Autodesk Fusion 360 part; units mm, degrees
note: some values were not read from the file. Set by a fixed rule: which face or edge a step refers to.
(part 5 of 20)
  spline S25 degree 5 poles (11.0419, -11.5792) (11.0412, -11.5772) (11.0398, -11.5731) (11.0377, -11.5671) (11.035, -11.5591) (11.0315, -11.5491) (11.028, -11.5391) (11.0246, -11.5291) (11.0211, -11.5192) (11.0176, -11.5093) (11.0141, -11.4995) (11.0106, -11.4897) (11.0071, -11.4799) (11.0036, -11.4701) (11.0001, -11.4604) (10.9966, -11.4507) (10.993, -11.441) (10.9895, -11.4313) (10.986, -11.4217) (10.9824, -11.4122) (10.9789, -11.4026) (10.9753, -11.3931) (10.9717, -11.3836) (10.9682, -11.3742) (10.9646, -11.3647) (10.961, -11.3553) (10.9574, -11.346) (10.9538, -11.3367) (10.9502, -11.3274) (10.9466, -11.3181) (10.943, -11.3089) (10.9394, -11.2997) (10.9358, -11.2905) (10.9321, -11.2814) (10.9285, -11.2723) (10.9249, -11.2632) (10.9212, -11.2541) (10.9176, -11.2451) (10.9139, -11.2362) (10.9103, -11.2272) (10.9066, -11.2183) (10.903, -11.2094) (10.8993, -11.2006) (10.8957, -11.1918) (10.892, -11.183) (10.8883, -11.1743) (10.8847, -11.1655) (10.881, -11.1569) (10.8773, -11.1482) (10.8736, -11.1396) (10.8699, -11.131) (10.8662, -11.1225) (10.8625, -11.114) (10.8589, -11.1055) (10.8552, -11.097) (10.8515, -11.0886) (10.8478, -11.0803) (10.8441, -11.0719) (10.8404, -11.0636) (10.8367, -11.0553) (10.833, -11.0471) (10.8292, -11.0389) (10.8255, -11.0307) (10.8218, -11.0226) (10.8181, -11.0145) (10.8144, -11.0064) (10.8107, -10.9984) (10.807, -10.9903) (10.8033, -10.9824) (10.7996, -10.9745) (10.7958, -10.9666) (10.7921, -10.9587) (10.7884, -10.9509) (10.7847, -10.9431) (10.781, -10.9353) (10.7773, -10.9276) (10.7736, -10.9199) (10.7699, -10.9123) (10.7662, -10.9046) (10.7625, -10.8971) (10.7587, -10.8895) (10.755, -10.882) (10.7513, -10.8745) (10.7476, -10.8671) (10.7439, -10.8597) (10.7402, -10.8523) (10.7365, -10.845) (10.7328, -10.8377) (10.7292, -10.8305) (10.7255, -10.8233) (10.7218, -10.8161) (10.7181, -10.8089) (10.7144, -10.8018) (10.7107, -10.7947) (10.7071, -10.7877) (10.7034, -10.7807) (10.6997, -10.7738) (10.6961, -10.7668) (10.6924, -10.7599) (10.6888, -10.7531) (10.6851, -10.7463) (10.6815, -10.7395) (10.6778, -10.7328) (10.6742, -10.7261) (10.6706, -10.7194) (10.6669, -10.7128) (10.6633, -10.7062) (10.6597, -10.6997) (10.6561, -10.6931) (10.6525, -10.6867) (10.6489, -10.6802) (10.6453, -10.6738) (10.6417, -10.6675) (10.6381, -10.6612) (10.6346, -10.6549) (10.631, -10.6487) (10.6275, -10.6425) (10.6239, -10.6363) (10.6204, -10.6302) (10.6168, -10.6241) (10.6133, -10.618) (10.6098, -10.612) (10.6063, -10.6061) (10.6028, -10.6001) (10.5993, -10.5943) (10.5958, -10.5884) (10.5923, -10.5826) (10.5889, -10.5768) (10.5854, -10.5711) (10.582, -10.5654) (10.5785, -10.5598) (10.5751, -10.5542) (10.5717, -10.5486) (10.5683, -10.5431) (10.5649, -10.5376) (10.5615, -10.5321) (10.5582, -10.5267) (10.5548, -10.5214) (10.5515, -10.516) (10.5481, -10.5108) (10.5448, -10.5055) (10.5415, -10.5003) (10.5382, -10.4952) (10.5349, -10.4901) (10.5316, -10.485) (10.5284, -10.48) (10.5251, -10.475) (10.5219, -10.47) (10.5187, -10.4651) (10.5155, -10.4603) (10.5123, -10.4554) (10.5091, -10.4507) (10.506, -10.4459) (10.5028, -10.4412) (10.4997, -10.4366) (10.4966, -10.432) (10.4935, -10.4274) (10.4904, -10.4229) (10.4874, -10.4184) (10.4843, -10.414) (10.4813, -10.4096) (10.4783, -10.4052) (10.4753, -10.4009) (10.4723, -10.3967) (10.4694, -10.3925) (10.4664, -10.3883) (10.4635, -10.3842) (10.4606, -10.3801) (10.4577, -10.376) (10.4549, -10.3721) (10.452, -10.3681) (10.4492, -10.3642) (10.4464, -10.3603) (10.4436, -10.3565) (10.4409, -10.3528) (10.4382, -10.349) (10.4354, -10.3454) (10.4328, -10.3417) (10.4301, -10.3382) (10.4274, -10.3346) (10.4248, -10.3311) (10.4222, -10.3277) (10.4197, -10.3243) (10.4171, -10.3209) (10.4146, -10.3176) (10.4121, -10.3144) (10.4096, -10.3112) (10.4072, -10.308) (10.4048, -10.3049) (10.4024, -10.3018) (10.4, -10.2988) (10.3977, -10.2958) (10.3954, -10.2929) (10.3931, -10.29) (10.3908, -10.2872) (10.3886, -10.2844) (10.3864, -10.2817) (10.3842, -10.279) (10.3821, -10.2764) (10.38, -10.2738) (10.3779, -10.2712) (10.3759, -10.2688) (10.3739, -10.2663) (10.3719, -10.2639) (10.37, -10.2616) (10.368, -10.2593) (10.3662, -10.2571) (10.3643, -10.2549) (10.3625, -10.2528) (10.3608, -10.2507) (10.359, -10.2486) (10.3573, -10.2467) (10.3557, -10.2447) (10.354, -10.2429) (10.3525, -10.241) (10.3509, -10.2393) (10.3494, -10.2376) (10.3479, -10.2359) (10.3465, -10.2343) (10.3451, -10.2327) (10.3438, -10.2312) (10.3425, -10.2298) (10.3412, -10.2284) (10.34, -10.227) (10.3388, -10.2257) (10.3377, -10.2245) (10.3366, -10.2233) (10.3356, -10.2222) (10.3346, -10.2211) (10.3336, -10.2201) (10.3327, -10.2191) (10.3319, -10.2182) (10.3311, -10.2174) (10.3303, -10.2166) (10.3296, -10.2159) (10.329, -10.2152) (10.3284, -10.2146) (10.3279, -10.214) (10.3274, -10.2135) (10.3269, -10.2131) (10.3266, -10.2127) (10.3263, -10.2124) (10.3261, -10.2123) (10.326, -10.2122) (10.326, -10.2121) knots -1 -1 -1 -1 -1 -1 -0.99583333 -0.99166667 -0.9875 -0.98333333 -0.97916667 -0.975 -0.97083333 -0.96666667 -0.9625 -0.95833333 -0.95416667 -0.95 -0.94583333 -0.94166667 -0.9375 -0.93333333 -0.92916667 -0.925 -0.92083333 -0.91666667 -0.9125 -0.90833333 -0.90416667 -0.9 -0.89583333 -0.89166667 -0.8875 -0.88333333 -0.87916667 -0.875 -0.87083333 -0.86666667 -0.8625 -0.85833333 -0.85416667 -0.85 -0.84583333 -0.84166667 -0.8375 -0.83333333 -0.82916667 -0.825 -0.82083333 -0.81666667 -0.8125 -0.80833333 -0.80416667 -0.8 -0.79583333 -0.79166667 -0.7875 -0.78333333 -0.77916667 -0.775 -0.77083333 -0.76666667 -0.7625 -0.75833333 -0.75416667 -0.75 -0.74583333 -0.74166667 -0.7375 -0.73333333 -0.72916667 -0.725 -0.72083333 -0.71666667 -0.7125 -0.70833333 -0.70416667 -0.7 -0.69583333 -0.69166667 -0.6875 -0.68333333 -0.67916667 -0.675 -0.67083333 -0.66666667 -0.6625 -0.65833333 -0.65416667 -0.65 -0.64583333 -0.64166667 -0.6375 -0.63333333 -0.62916667 -0.625 -0.62083333 -0.61666667 -0.6125 -0.60833333 -0.60416667 -0.6 -0.59583333 -0.59166667 -0.5875 -0.58333333 -0.57916667 -0.575 -0.57083333 -0.56666667 -0.5625 -0.55833333 -0.55416667 -0.55 -0.54583333 -0.54166667 -0.5375 -0.53333333 -0.52916667 -0.525 -0.52083333 -0.51666667 -0.5125 -0.50833333 -0.50416667 -0.5 -0.49583333 -0.49166667 -0.4875 -0.48333333 -0.47916667 -0.475 -0.47083333 -0.46666667 -0.4625 -0.45833333 -0.45416667 -0.45 -0.44583333 -0.44166667 -0.4375 -0.43333333 -0.42916667 -0.425 -0.42083333 -0.41666667 -0.4125 -0.40833333 -0.40416667 -0.4 -0.39583333 -0.39166667 -0.3875 -0.38333333 -0.37916667 -0.375 -0.37083333 -0.36666667 -0.3625 -0.35833333 -0.35416667 -0.35 -0.34583333 -0.34166667 -0.3375 -0.33333333 -0.32916667 -0.325 -0.32083333 -0.31666667 -0.3125 -0.30833333 -0.30416667 -0.3 -0.29583333 -0.29166667 -0.2875 -0.28333333 -0.27916667 -0.275 -0.27083333 -0.26666667 -0.2625 -0.25833333 -0.25416667 -0.25 -0.24583333 -0.24166667 -0.2375 -0.23333333 -0.22916667 -0.225 -0.22083333 -0.21666667 -0.2125 -0.20833333 -0.20416667 -0.2 -0.19583333 -0.19166667 -0.1875 -0.18333333 -0.17916667 -0.175 -0.17083333 -0.16666667 -0.1625 -0.15833333 -0.15416667 -0.15 -0.14583333 -0.14166667 -0.1375 -0.13333333 -0.12916667 -0.125 -0.12083333 -0.11666667 -0.1125 -0.10833333 -0.10416667 -0.1 -0.09583333 -0.09166667 -0.0875 -0.08333333 -0.07916667 -0.075 -0.07083333 -0.06666667 -0.0625 -0.05833333 -0.05416667 -0.05 -0.04583333 -0.04166667 -0.0375 -0.03333333 -0.02916667 -0.025 -0.02083333 -0.01666667 -0.0125 -0.00833333 -0.00416667 0 0 0 0 0 0
  spline S26 degree 5 poles (9.0768, -11.3369) (9.0769, -11.3369) (9.0769, -11.337) (9.0771, -11.3372) (9.0773, -11.3375) (9.0777, -11.3379) (9.0781, -11.3384) (9.0785, -11.3389) (9.079, -11.3395) (9.0796, -11.3402) (9.0802, -11.3409) (9.0808, -11.3417) (9.0815, -11.3425) (9.0823, -11.3434) (9.0831, -11.3443) (9.084, -11.3453) (9.0849, -11.3464) (9.0858, -11.3475) (9.0868, -11.3486) (9.0879, -11.3498) (9.089, -11.3511) (9.0902, -11.3524) (9.0914, -11.3537) (9.0926, -11.3551) (9.0939, -11.3566) (9.0953, -11.3581) (9.0967, -11.3596) (9.0982, -11.3612) (9.0997, -11.3628) (9.1012, -11.3645) (9.1028, -11.3662) (9.1045, -11.368) (9.1062, -11.3698) (9.1079, -11.3717) (9.1097, -11.3735) (9.1115, -11.3755) (9.1134, -11.3775) (9.1153, -11.3795) (9.1173, -11.3815) (9.1194, -11.3836) (9.1214, -11.3858) (9.1235, -11.388) (9.1257, -11.3902) (9.1279, -11.3924) (9.1302, -11.3947) (9.1325, -11.397) (9.1348, -11.3994) (9.1372, -11.4018) (9.1397, -11.4042) (9.1422, -11.4067) (9.1447, -11.4092) (9.1473, -11.4117) (9.1499, -11.4143) (9.1526, -11.4169) (9.1553, -11.4195) (9.158, -11.4222) (9.1608, -11.4249) (9.1637, -11.4276) (9.1666, -11.4304) (9.1695, -11.4332) (9.1725, -11.436) (9.1755, -11.4389) (9.1786, -11.4418) (9.1817, -11.4447) (9.1848, -11.4476) (9.188, -11.4506) (9.1913, -11.4536) (9.1946, -11.4566) (9.1979, -11.4597) (9.2013, -11.4627) (9.2047, -11.4658) (9.2081, -11.469) (9.2116, -11.4721) (9.2152, -11.4753) (9.2188, -11.4785) (9.2224, -11.4818) (9.2261, -11.485) (9.2298, -11.4883) (9.2335, -11.4916) (9.2373, -11.495) (9.2412, -11.4983) (9.2451, -11.5017) (9.249, -11.5051) (9.253, -11.5085) (9.257, -11.512) (9.261, -11.5154) (9.2651, -11.5189) (9.2692, -11.5224) (9.2734, -11.526) (9.2776, -11.5295) (9.2819, -11.5331) (9.2862, -11.5367) (9.2905, -11.5403) (9.2949, -11.544) (9.2993, -11.5476) (9.3038, -11.5513) (9.3083, -11.555) (9.3128, -11.5587) (9.3174, -11.5624) (9.322, -11.5662) (9.3267, -11.5699) (9.3314, -11.5737) (9.3361, -11.5775) (9.3409, -11.5813) (9.3457, -11.5852) (9.3506, -11.589) (9.3555, -11.5929) (9.3605, -11.5968) (9.3654, -11.6007) (9.3705, -11.6046) (9.3755, -11.6085) (9.3806, -11.6125) (9.3858, -11.6164) (9.3909, -11.6204) (9.3962, -11.6244) (9.4014, -11.6284) (9.4067, -11.6324) (9.412, -11.6365) (9.4174, -11.6405) (9.4228, -11.6446) (9.4283, -11.6486) (9.4338, -11.6527) (9.4393, -11.6568) (9.4449, -11.6609) (9.4505, -11.6651) (9.4561, -11.6692) (9.4618, -11.6733) (9.4675, -11.6775) (9.4733, -11.6817) (9.4791, -11.6859) (9.4849, -11.6901) (9.4908, -11.6943) (9.4967, -11.6985) (9.5026, -11.7027) (9.5086, -11.707) (9.5146, -11.7112) (9.5207, -11.7155) (9.5268, -11.7197) (9.5329, -11.724) (9.5391, -11.7283) (9.5453, -11.7326) (9.5516, -11.7369) (9.5578, -11.7412) (9.5642, -11.7455) (9.5705, -11.7499) (9.5769, -11.7542) (9.5833, -11.7586) (9.5898, -11.7629) (9.5963, -11.7673) (9.6028, -11.7717) (9.6094, -11.776) (9.616, -11.7804) (9.6227, -11.7848) (9.6294, -11.7892) (9.6361, -11.7936) (9.6428, -11.798) (9.6496, -11.8025) (9.6565, -11.8069) (9.6633, -11.8113) (9.6702, -11.8158) (9.6772, -11.8202) (9.6841, -11.8247) (9.6912, -11.8291) (9.6982, -11.8336) (9.7053, -11.8381) (9.7124, -11.8425) (9.7195, -11.847) (9.7267, -11.8515) (9.7339, -11.856) (9.7412, -11.8605) (9.7485, -11.865) (9.7558, -11.8695) (9.7632, -11.874) (9.7706, -11.8785) (9.778, -11.883) (9.7855, -11.8875) (9.793, -11.8921) (9.8005, -11.8966) (9.8081, -11.9011) (9.8157, -11.9056) (9.8233, -11.9102) (9.831, -11.9147) (9.8387, -11.9193) (9.8464, -11.9238) (9.8542, -11.9283) (9.862, -11.9329) (9.8699, -11.9374) (9.8777, -11.942) (9.8857, -11.9465) (9.8936, -11.9511) (9.9016, -11.9557) (9.9096, -11.9602) (9.9176, -11.9648) (9.9257, -11.9693) (9.9338, -11.9739) (9.942, -11.9785) (9.9502, -11.983) (9.9584, -11.9876) (9.9666, -11.9921) (9.9749, -11.9967) (9.9832, -12.0013) (9.9916, -12.0058) (9.9999, -12.0104) (10.0084, -12.015) (10.0168, -12.0195) (10.0253, -12.0241) (10.0338, -12.0287) (10.0423, -12.0332) (10.0509, -12.0378) (10.0595, -12.0423) (10.0682, -12.0469) (10.0768, -12.0515) (10.0855, -12.056) (10.0943, -12.0606) (10.1031, -12.0651) (10.1119, -12.0697) (10.1207, -12.0743) (10.1296, -12.0788) (10.1385, -12.0834) (10.1474, -12.0879) (10.1564, -12.0924) (10.1654, -12.097) (10.1744, -12.1015) (10.1834, -12.1061) (10.1925, -12.1106) (10.2017, -12.1151) (10.2108, -12.1197) (10.22, -12.1242) (10.2292, -12.1287) (10.2385, -12.1332) (10.2478, -12.1378) (10.2571, -12.1423) (10.2664, -12.1468) (10.2758, -12.1513) (10.2852, -12.1558) (10.2946, -12.1603) (10.3041, -12.1648) (10.3136, -12.1693) (10.3231, -12.1738) (10.3327, -12.1783) (10.3423, -12.1828) (10.35, -12.1863) (10.3558, -12.189) (10.3596, -12.1908) (10.3616, -12.1917) knots 0 0 0 0 0 0 0.00416667 0.00833333 0.0125 0.01666667 0.02083333 0.025 0.02916667 0.03333333 0.0375 0.04166667 0.04583333 0.05 0.05416667 0.05833333 0.0625 0.06666667 0.07083333 0.075 0.07916667 0.08333333 0.0875 0.09166667 0.09583333 0.1 0.10416667 0.10833333 0.1125 0.11666667 0.12083333 0.125 0.12916667 0.13333333 0.1375 0.14166667 0.14583333 0.15 0.15416667 0.15833333 0.1625 0.16666667 0.17083333 0.175 0.17916667 0.18333333 0.1875 0.19166667 0.19583333 0.2 0.20416667 0.20833333 0.2125 0.21666667 0.22083333 0.225 0.22916667 0.23333333 0.2375 0.24166667 0.24583333 0.25 0.25416667 0.25833333 0.2625 0.26666667 0.27083333 0.275 0.27916667 0.28333333 0.2875 0.29166667 0.29583333 0.3 0.30416667 0.30833333 0.3125 0.31666667 0.32083333 0.325 0.32916667 0.33333333 0.3375 0.34166667 0.34583333 0.35 0.35416667 0.35833333 0.3625 0.36666667 0.37083333 0.375 0.37916667 0.38333333 0.3875 0.39166667 0.39583333 0.4 0.40416667 0.40833333 0.4125 0.41666667 0.42083333 0.425 0.42916667 0.43333333 0.4375 0.44166667 0.44583333 0.45 0.45416667 0.45833333 0.4625 0.46666667 0.47083333 0.475 0.47916667 0.48333333 0.4875 0.49166667 0.49583333 0.5 0.50416667 0.50833333 0.5125 0.51666667 0.52083333 0.525 0.52916667 0.53333333 0.5375 0.54166667 0.54583333 0.55 0.55416667 0.55833333 0.5625 0.56666667 0.57083333 0.575 0.57916667 0.58333333 0.5875 0.59166667 0.59583333 0.6 0.60416667 0.60833333 0.6125 0.61666667 0.62083333 0.625 0.62916667 0.63333333 0.6375 0.64166667 0.64583333 0.65 0.65416667 0.65833333 0.6625 0.66666667 0.67083333 0.675 0.67916667 0.68333333 0.6875 0.69166667 0.69583333 0.7 0.70416667 0.70833333 0.7125 0.71666667 0.72083333 0.725 0.72916667 0.73333333 0.7375 0.74166667 0.74583333 0.75 0.75416667 0.75833333 0.7625 0.76666667 0.77083333 0.775 0.77916667 0.78333333 0.7875 0.79166667 0.79583333 0.8 0.80416667 0.80833333 0.8125 0.81666667 0.82083333 0.825 0.82916667 0.83333333 0.8375 0.84166667 0.84583333 0.85 0.85416667 0.85833333 0.8625 0.86666667 0.87083333 0.875 0.87916667 0.88333333 0.8875 0.89166667 0.89583333 0.9 0.90416667 0.90833333 0.9125 0.91666667 0.92083333 0.925 0.92916667 0.93333333 0.9375 0.94166667 0.94583333 0.95 0.95416667 0.95833333 0.9625 0.96666667 0.97083333 0.975 0.97916667 0.98333333 0.9875 0.99166667 0.99583333 1 1 1 1 1 1
  line L50 (-11.5731, -7.4247) -> (-12.223, -7.8417)
  arc A40 (-12.2165, -6.3102) -> (-11.5731, -7.4247) centre (0, 0) ccw
  line L51 (11.235, -9.2016) -> (11.2355, -9.202)
  line L52 (10.6376, -8.7123) -> (11.235, -9.2016)
  line L53 (10.3255, -10.2117) -> (9.7765, -9.6687)
  spline S27 degree 5 poles (-14.4246, -6.9233) (-14.4224, -6.9232) (-14.4182, -6.9232) (-14.4118, -6.9231) (-14.4033, -6.9229) (-14.3927, -6.9227) (-14.3822, -6.9225) (-14.3716, -6.9223) (-14.3611, -6.9221) (-14.3507, -6.9218) (-14.3402, -6.9215) (-14.3298, -6.9212) (-14.3194, -6.9209) (-14.309, -6.9206) (-14.2987, -6.9203) (-14.2883, -6.9199) (-14.2781, -6.9195) (-14.2678, -6.9192) (-14.2576, -6.9188) (-14.2474, -6.9183) (-14.2372, -6.9179) (-14.227, -6.9175) (-14.2169, -6.917) (-14.2068, -6.9165) (-14.1967, -6.916) (-14.1867, -6.9155) (-14.1767, -6.915) (-14.1667, -6.9145) (-14.1568, -6.9139) (-14.1468, -6.9134) (-14.1369, -6.9128) (-14.1271, -6.9122) (-14.1172, -6.9116) (-14.1074, -6.9109) (-14.0976, -6.9103) (-14.0879, -6.9097) (-14.0782, -6.909) (-14.0685, -6.9083) (-14.0588, -6.9076) (-14.0492, -6.9069) (-14.0396, -6.9062) (-14.03, -6.9055) (-14.0205, -6.9047) (-14.011, -6.9039) (-14.0015, -6.9032) (-13.992, -6.9024) (-13.9826, -6.9016) (-13.9732, -6.9008) (-13.9639, -6.8999) (-13.9545, -6.8991) (-13.9452, -6.8982) (-13.936, -6.8974) (-13.9267, -6.8965) (-13.9175, -6.8956) (-13.9083, -6.8947) (-13.8992, -6.8938) (-13.8901, -6.8929) (-13.881, -6.8919) (-13.872, -6.891) (-13.8629, -6.89) (-13.854, -6.889) (-13.845, -6.888) (-13.8361, -6.887) (-13.8272, -6.886) (-13.8184, -6.885) (-13.8095, -6.884) (-13.8007, -6.8829) (-13.792, -6.8818) (-13.7833, -6.8808) (-13.7746, -6.8797) (-13.7659, -6.8786) (-13.7573, -6.8775) (-13.7487, -6.8764) (-13.7401, -6.8753) (-13.7316, -6.8741) (-13.7231, -6.873) (-13.7147, -6.8718) (-13.7063, -6.8707) (-13.6979, -6.8695) (-13.6895, -6.8683) (-13.6812, -6.8671) (-13.6729, -6.8659) (-13.6647, -6.8647) (-13.6564, -6.8635) (-13.6483, -6.8623) (-13.6401, -6.861) (-13.632, -6.8598) (-13.6239, -6.8585) (-13.6159, -6.8572) (-13.6079, -6.856) (-13.5999, -6.8547) (-13.592, -6.8534) (-13.5841, -6.8521) (-13.5762, -6.8508) (-13.5684, -6.8494) (-13.5606, -6.8481) (-13.5528, -6.8468) (-13.5451, -6.8454) (-13.5375, -6.8441) (-13.5298, -6.8427) (-13.5222, -6.8414) (-13.5146, -6.84) (-13.5071, -6.8386) (-13.4996, -6.8372) (-13.4922, -6.8358) (-13.4847, -6.8344) (-13.4773, -6.833) (-13.47, -6.8316) (-13.4627, -6.8302) (-13.4554, -6.8288) (-13.4482, -6.8273) (-13.441, -6.8259) (-13.4339, -6.8244) (-13.4267, -6.823) (-13.4197, -6.8215) (-13.4126, -6.8201) (-13.4056, -6.8186) (-13.3987, -6.8171) (-13.3918, -6.8157) (-13.3849, -6.8142) (-13.378, -6.8127) (-13.3712, -6.8112) (-13.3645, -6.8097) (-13.3578, -6.8082) (-13.3511, -6.8067) (-13.3445, -6.8052) (-13.3379, -6.8037) (-13.3313, -6.8022) (-13.3248, -6.8007) (-13.3183, -6.7992) (-13.3119, -6.7976) (-13.3055, -6.7961) (-13.2991, -6.7946) (-13.2928, -6.7931) (-13.2866, -6.7915) (-13.2804, -6.79) (-13.2742, -6.7885) (-13.268, -6.7869) (-13.2619, -6.7854) (-13.2559, -6.7839) (-13.2499, -6.7823) (-13.2439, -6.7808) (-13.238, -6.7792) (-13.2321, -6.7777) (-13.2263, -6.7761) (-13.2205, -6.7746) (-13.2147, -6.7731) (-13.209, -6.7715) (-13.2034, -6.77) (-13.1978, -6.7684) (-13.1922, -6.7669) (-13.1867, -6.7653) (-13.1812, -6.7638) (-13.1758, -6.7623) (-13.1704, -6.7607) (-13.165, -6.7592) (-13.1597, -6.7577) (-13.1545, -6.7561) (-13.1493, -6.7546) (-13.1441, -6.7531) (-13.139, -6.7516) (-13.1339, -6.75) (-13.1289, -6.7485) (-13.124, -6.747) (-13.119, -6.7455) (-13.1142, -6.744) (-13.1093, -6.7425) (-13.1046, -6.741) (-13.0998, -6.7395) (-13.0951, -6.738) (-13.0905, -6.7366) (-13.0859, -6.7351) (-13.0814, -6.7336) (-13.0769, -6.7321) (-13.0725, -6.7307) (-13.0681, -6.7292) (-13.0638, -6.7278) (-13.0595, -6.7264) (-13.0552, -6.7249) (-13.0511, -6.7235) (-13.0469, -6.7221) (-13.0429, -6.7207) (-13.0388, -6.7193) (-13.0349, -6.7179) (-13.0309, -6.7165) (-13.0271, -6.7152) (-13.0232, -6.7138) (-13.0195, -6.7125) (-13.0158, -6.7111) (-13.0121, -6.7098) (-13.0085, -6.7085) (-13.005, -6.7072) (-13.0015, -6.7059) (-12.998, -6.7046) (-12.9946, -6.7033) (-12.9913, -6.7021) (-12.988, -6.7008) (-12.9848, -6.6996) (-12.9816, -6.6984) (-12.9785, -6.6972) (-12.9755, -6.696) (-12.9725, -6.6948) (-12.9695, -6.6937) (-12.9667, -6.6925) (-12.9638, -6.6914) (-12.9611, -6.6903) (-12.9584, -6.6892) (-12.9557, -6.6881) (-12.9531, -6.6871) (-12.9506, -6.686) (-12.9482, -6.685) (-12.9457, -6.684) (-12.9434, -6.683) (-12.9411, -6.6821) (-12.9389, -6.6811) (-12.9367, -6.6802) (-12.9346, -6.6793) (-12.9326, -6.6784) (-12.9306, -6.6775) (-12.9287, -6.6767) (-12.9269, -6.6759) (-12.9251, -6.6751) (-12.9234, -6.6743) (-12.9217, -6.6736) (-12.9201, -6.6729) (-12.9186, -6.6722) (-12.9171, -6.6715) (-12.9157, -6.6709) (-12.9144, -6.6703) (-12.9132, -6.6697) (-12.912, -6.6691) (-12.9108, -6.6686) (-12.9098, -6.6681) (-12.9088, -6.6676) (-12.9079, -6.6672) (-12.9071, -6.6668) (-12.9063, -6.6664) (-12.9056, -6.6661) (-12.905, -6.6658) (-12.9044, -6.6655) (-12.9039, -6.6652) (-12.9036, -6.6651) (-12.9034, -6.665) (-12.9033, -6.6649) (-12.9032, -6.6649) knots -1 -1 -1 -1 -1 -1 -0.99583333 -0.99166667 -0.9875 -0.98333333 -0.97916667 -0.975 -0.97083333 -0.96666667 -0.9625 -0.95833333 -0.95416667 -0.95 -0.94583333 -0.94166667 -0.9375 -0.93333333 -0.92916667 -0.925 -0.92083333 -0.91666667 -0.9125 -0.90833333 -0.90416667 -0.9 -0.89583333 -0.89166667 -0.8875 -0.88333333 -0.87916667 -0.875 -0.87083333 -0.86666667 -0.8625 -0.85833333 -0.85416667 -0.85 -0.84583333 -0.84166667 -0.8375 -0.83333333 -0.82916667 -0.825 -0.82083333 -0.81666667 -0.8125 -0.80833333 -0.80416667 -0.8 -0.79583333 -0.79166667 -0.7875 -0.78333333 -0.77916667 -0.775 -0.77083333 -0.76666667 -0.7625 -0.75833333 -0.75416667 -0.75 -0.74583333 -0.74166667 -0.7375 -0.73333333 -0.72916667 -0.725 -0.72083333 -0.71666667 -0.7125 -0.70833333 -0.70416667 -0.7 -0.69583333 -0.69166667 -0.6875 -0.68333333 -0.67916667 -0.675 -0.67083333 -0.66666667 -0.6625 -0.65833333 -0.65416667 -0.65 -0.64583333 -0.64166667 -0.6375 -0.63333333 -0.62916667 -0.625 -0.62083333 -0.61666667 -0.6125 -0.60833333 -0.60416667 -0.6 -0.59583333 -0.59166667 -0.5875 -0.58333333 -0.57916667 -0.575 -0.57083333 -0.56666667 -0.5625 -0.55833333 -0.55416667 -0.55 -0.54583333 -0.54166667 -0.5375 -0.53333333 -0.52916667 -0.525 -0.52083333 -0.51666667 -0.5125 -0.50833333 -0.50416667 -0.5 -0.49583333 -0.49166667 -0.4875 -0.48333333 -0.47916667 -0.475 -0.47083333 -0.46666667 -0.4625 -0.45833333 -0.45416667 -0.45 -0.44583333 -0.44166667 -0.4375 -0.43333333 -0.42916667 -0.425 -0.42083333 -0.41666667 -0.4125 -0.40833333 -0.40416667 -0.4 -0.39583333 -0.39166667 -0.3875 -0.38333333 -0.37916667 -0.375 -0.37083333 -0.36666667 -0.3625 -0.35833333 -0.35416667 -0.35 -0.34583333 -0.34166667 -0.3375 -0.33333333 -0.32916667 -0.325 -0.32083333 -0.31666667 -0.3125 -0.30833333 -0.30416667 -0.3 -0.29583333 -0.29166667 -0.2875 -0.28333333 -0.27916667 -0.275 -0.27083333 -0.26666667 -0.2625 -0.25833333 -0.25416667 -0.25 -0.24583333 -0.24166667 -0.2375 -0.23333333 -0.22916667 -0.225 -0.22083333 -0.21666667 -0.2125 -0.20833333 -0.20416667 -0.2 -0.19583333 -0.19166667 -0.1875 -0.18333333 -0.17916667 -0.175 -0.17083333 -0.16666667 -0.1625 -0.15833333 -0.15416667 -0.15 -0.14583333 -0.14166667 -0.1375 -0.13333333 -0.12916667 -0.125 -0.12083333 -0.11666667 -0.1125 -0.10833333 -0.10416667 -0.1 -0.09583333 -0.09166667 -0.0875 -0.08333333 -0.07916667 -0.075 -0.07083333 -0.06666667 -0.0625 -0.05833333 -0.05416667 -0.05 -0.04583333 -0.04166667 -0.0375 -0.03333333 -0.02916667 -0.025 -0.02083333 -0.01666667 -0.0125 -0.00833333 -0.00416667 0 0 0 0 0 0
  arc A41 (9.7765, -9.6687) -> (10.6376, -8.7123) centre (0, 0) ccw
  spline S28 degree 5 poles (13.208, -9.0304) (13.2069, -9.0286) (13.2047, -9.0249) (13.2015, -9.0195) (13.1971, -9.0122) (13.1916, -9.0031) (13.1862, -8.9941) (13.1807, -8.9851) (13.1752, -8.9761) (13.1698, -8.9671) (13.1643, -8.9582) (13.1589, -8.9493) (13.1534, -8.9405) (13.1479, -8.9317) (13.1425, -8.9229) (13.137, -8.9141) (13.1315, -8.9054) (13.1261, -8.8967) (13.1206, -8.888) (13.1151, -8.8794) (13.1097, -8.8708) (13.1042, -8.8622) (13.0988, -8.8537) (13.0933, -8.8452) (13.0878, -8.8367) (13.0824, -8.8283) (13.0769, -8.8199) (13.0715, -8.8115) (13.066, -8.8032) (13.0606, -8.7948) (13.0551, -8.7866) (13.0497, -8.7783) (13.0442, -8.7701) (13.0388, -8.7619) (13.0333, -8.7538) (13.0279, -8.7456) (13.0224, -8.7376) (13.017, -8.7295) (13.0116, -8.7215) (13.0062, -8.7135) (13.0007, -8.7055) (12.9953, -8.6976) (12.9899, -8.6897) (12.9845, -8.6819) (12.9791, -8.6741) (12.9736, -8.6663) (12.9682, -8.6585) (12.9628, -8.6508) (12.9574, -8.6431) (12.9521, -8.6354) (12.9467, -8.6278) (12.9413, -8.6202) (12.9359, -8.6126) (12.9305, -8.6051) (12.9252, -8.5976) (12.9198, -8.5902) (12.9144, -8.5827) (12.9091, -8.5754) (12.9037, -8.568) (12.8984, -8.5607) (12.893, -8.5534) (12.8877, -8.5461) (12.8824, -8.5389) (12.8771, -8.5317) (12.8718, -8.5246) (12.8664, -8.5174) (12.8611, -8.5103) (12.8558, -8.5033) (12.8506, -8.4963) (12.8453, -8.4893) (12.84, -8.4823) (12.8347, -8.4754) (12.8295, -8.4685) (12.8242, -8.4617) (12.819, -8.4549) (12.8138, -8.4481) (12.8085, -8.4413) (12.8033, -8.4346) (12.7981, -8.4279) (12.7929, -8.4213) (12.7877, -8.4147) (12.7825, -8.4081) (12.7773, -8.4016) (12.7722, -8.3951) (12.767, -8.3886) (12.7619, -8.3822) (12.7567, -8.3758) (12.7516, -8.3694) (12.7465, -8.3631) (12.7414, -8.3568) (12.7363, -8.3505) (12.7312, -8.3443) (12.7261, -8.3381) (12.721, -8.332) (12.716, -8.3259) (12.7109, -8.3198) (12.7059, -8.3137) (12.7009, -8.3077) (12.6959, -8.3017) (12.6909, -8.2958) (12.6859, -8.2899) (12.6809, -8.284) (12.676, -8.2782) (12.671, -8.2724) (12.6661, -8.2666) (12.6612, -8.2609) (12.6562, -8.2552) (12.6513, -8.2496) (12.6465, -8.2439) (12.6416, -8.2384) (12.6367, -8.2328) (12.6319, -8.2273) (12.6271, -8.2218) (12.6223, -8.2164) (12.6175, -8.211) (12.6127, -8.2056) (12.6079, -8.2003) (12.6032, -8.195) (12.5984, -8.1898) (12.5937, -8.1846) (12.589, -8.1794) (12.5843, -8.1742) (12.5796, -8.1691) (12.575, -8.1641) (12.5703, -8.159) (12.5657, -8.154) (12.5611, -8.1491) (12.5565, -8.1441) (12.552, -8.1393) (12.5474, -8.1344) (12.5429, -8.1296) (12.5384, -8.1248) (12.5339, -8.1201) (12.5294, -8.1154) (12.5249, -8.1107) (12.5205, -8.1061) (12.5161, -8.1015) (12.5117, -8.097) (12.5073, -8.0925) (12.5029, -8.088) (12.4986, -8.0836) (12.4943, -8.0792) (12.49, -8.0748) (12.4857, -8.0705) (12.4815, -8.0662) (12.4772, -8.062) (12.473, -8.0578) (12.4688, -8.0536) (12.4647, -8.0495) (12.4605, -8.0454) (12.4564, -8.0413) (12.4523, -8.0373) (12.4482, -8.0333) (12.4442, -8.0294) (12.4401, -8.0255) (12.4361, -8.0216) (12.4322, -8.0178) (12.4282, -8.014) (12.4243, -8.0103) (12.4204, -8.0066) (12.4165, -8.0029) (12.4127, -7.9993) (12.4089, -7.9957) (12.4051, -7.9922) (12.4013, -7.9887) (12.3976, -7.9852) (12.3938, -7.9818) (12.3902, -7.9784) (12.3865, -7.975) (12.3829, -7.9717) (12.3793, -7.9684) (12.3757, -7.9652) (12.3722, -7.962) (12.3687, -7.9589) (12.3652, -7.9558) (12.3617, -7.9527) (12.3583, -7.9496) (12.3549, -7.9467) (12.3516, -7.9437) (12.3483, -7.9408) (12.345, -7.9379) (12.3417, -7.9351) (12.3385, -7.9323) (12.3353, -7.9296) (12.3322, -7.9268) (12.329, -7.9242) (12.326, -7.9216) (12.3229, -7.919) (12.3199, -7.9164) (12.3169, -7.9139) (12.314, -7.9115) (12.3111, -7.909) (12.3082, -7.9066) (12.3054, -7.9043) (12.3026, -7.902) (12.2998, -7.8998) (12.2971, -7.8975) (12.2944, -7.8954) (12.2918, -7.8932) (12.2892, -7.8911) (12.2867, -7.8891) (12.2841, -7.8871) (12.2817, -7.8851) (12.2792, -7.8832) (12.2769, -7.8813) (12.2745, -7.8795) (12.2722, -7.8777) (12.27, -7.8759) (12.2677, -7.8742) (12.2656, -7.8726) (12.2635, -7.8709) (12.2614, -7.8693) (12.2594, -7.8678) (12.2574, -7.8663) (12.2555, -7.8649) (12.2536, -7.8634) (12.2517, -7.8621) (12.25, -7.8608) (12.2482, -7.8595) (12.2465, -7.8582) (12.2449, -7.857) (12.2433, -7.8559) (12.2418, -7.8548) (12.2403, -7.8537) (12.2389, -7.8527) (12.2376, -7.8517) (12.2363, -7.8508) (12.235, -7.8499) (12.2338, -7.8491) (12.2327, -7.8483) (12.2316, -7.8475) (12.2306, -7.8468) (12.2296, -7.8462) (12.2287, -7.8455) (12.2279, -7.845) (12.2271, -7.8445) (12.2264, -7.844) (12.2258, -7.8435) (12.2252, -7.8431) (12.2247, -7.8428) (12.2242, -7.8425) (12.2239, -7.8423) (12.2237, -7.8422) (12.2236, -7.8421) (12.2236, -7.8421) knots -1 -1 -1 -1 -1 -1 -0.99583333 -0.99166667 -0.9875 -0.98333333 -0.97916667 -0.975 -0.97083333 -0.96666667 -0.9625 -0.95833333 -0.95416667 -0.95 -0.94583333 -0.94166667 -0.9375 -0.93333333 -0.92916667 -0.925 -0.92083333 -0.91666667 -0.9125 -0.90833333 -0.90416667 -0.9 -0.89583333 -0.89166667 -0.8875 -0.88333333 -0.87916667 -0.875 -0.87083333 -0.86666667 -0.8625 -0.85833333 -0.85416667 -0.85 -0.84583333 -0.84166667 -0.8375 -0.83333333 -0.82916667 -0.825 -0.82083333 -0.81666667 -0.8125 -0.80833333 -0.80416667 -0.8 -0.79583333 -0.79166667 -0.7875 -0.78333333 -0.77916667 -0.775 -0.77083333 -0.76666667 -0.7625 -0.75833333 -0.75416667 -0.75 -0.74583333 -0.74166667 -0.7375 -0.73333333 -0.72916667 -0.725 -0.72083333 -0.71666667 -0.7125 -0.70833333 -0.70416667 -0.7 -0.69583333 -0.69166667 -0.6875 -0.68333333 -0.67916667 -0.675 -0.67083333 -0.66666667 -0.6625 -0.65833333 -0.65416667 -0.65 -0.64583333 -0.64166667 -0.6375 -0.63333333 -0.62916667 -0.625 -0.62083333 -0.61666667 -0.6125 -0.60833333 -0.60416667 -0.6 -0.59583333 -0.59166667 -0.5875 -0.58333333 -0.57916667 -0.575 -0.57083333 -0.56666667 -0.5625 -0.55833333 -0.55416667 -0.55 -0.54583333 -0.54166667 -0.5375 -0.53333333 -0.52916667 -0.525 -0.52083333 -0.51666667 -0.5125 -0.50833333 -0.50416667 -0.5 -0.49583333 -0.49166667 -0.4875 -0.48333333 -0.47916667 -0.475 -0.47083333 -0.46666667 -0.4625 -0.45833333 -0.45416667 -0.45 -0.44583333 -0.44166667 -0.4375 -0.43333333 -0.42916667 -0.425 -0.42083333 -0.41666667 -0.4125 -0.40833333 -0.40416667 -0.4 -0.39583333 -0.39166667 -0.3875 -0.38333333 -0.37916667 -0.375 -0.37083333 -0.36666667 -0.3625 -0.35833333 -0.35416667 -0.35 -0.34583333 -0.34166667 -0.3375 -0.33333333 -0.32916667 -0.325 -0.32083333 -0.31666667 -0.3125 -0.30833333 -0.30416667 -0.3 -0.29583333 -0.29166667 -0.2875 -0.28333333 -0.27916667 -0.275 -0.27083333 -0.26666667 -0.2625 -0.25833333 -0.25416667 -0.25 -0.24583333 -0.24166667 -0.2375 -0.23333333 -0.22916667 -0.225 -0.22083333 -0.21666667 -0.2125 -0.20833333 -0.20416667 -0.2 -0.19583333 -0.19166667 -0.1875 -0.18333333 -0.17916667 -0.175 -0.17083333 -0.16666667 -0.1625 -0.15833333 -0.15416667 -0.15 -0.14583333 -0.14166667 -0.1375 -0.13333333 -0.12916667 -0.125 -0.12083333 -0.11666667 -0.1125 -0.10833333 -0.10416667 -0.1 -0.09583333 -0.09166667 -0.0875 -0.08333333 -0.07916667 -0.075 -0.07083333 -0.06666667 -0.0625 -0.05833333 -0.05416667 -0.05 -0.04583333 -0.04166667 -0.0375 -0.03333333 -0.02916667 -0.025 -0.02083333 -0.01666667 -0.0125 -0.00833333 -0.00416667 0 0 0 0 0 0
  arc A42 (12.6699, -9.771) -> (13.208, -9.0304) centre (0, 0) ccw
  spline S29 degree 5 poles (12.9032, -6.6649) (12.9033, -6.6649) (12.9034, -6.665) (12.9036, -6.6651) (12.9039, -6.6652) (12.9044, -6.6655) (12.905, -6.6658) (12.9056, -6.6661) (12.9063, -6.6664) (12.9071, -6.6668) (12.9079, -6.6672) (12.9088, -6.6676) (12.9098, -6.6681) (12.9108, -6.6686) (12.912, -6.6691) (12.9132, -6.6697) (12.9144, -6.6703) (12.9157, -6.6709) (12.9171, -6.6715) (12.9186, -6.6722) (12.9201, -6.6729) (12.9217, -6.6736) (12.9234, -6.6743) (12.9251, -6.6751) (12.9269, -6.6759) (12.9287, -6.6767) (12.9306, -6.6775) (12.9326, -6.6784) (12.9346, -6.6793) (12.9367, -6.6802) (12.9389, -6.6811) (12.9411, -6.6821) (12.9434, -6.683) (12.9457, -6.684) (12.9482, -6.685) (12.9506, -6.686) (12.9531, -6.6871) (12.9557, -6.6881) (12.9584, -6.6892) (12.9611, -6.6903) (12.9638, -6.6914) (12.9667, -6.6925) (12.9695, -6.6937) (12.9725, -6.6948) (12.9755, -6.696) (12.9785, -6.6972) (12.9816, -6.6984) (12.9848, -6.6996) (12.988, -6.7008) (12.9913, -6.7021) (12.9946, -6.7033) (12.998, -6.7046) (13.0015, -6.7059) (13.005, -6.7072) (13.0085, -6.7085) (13.0121, -6.7098) (13.0158, -6.7111) (13.0195, -6.7125) (13.0232, -6.7138) (13.0271, -6.7152) (13.0309, -6.7165) (13.0349, -6.7179) (13.0388, -6.7193) (13.0429, -6.7207) (13.0469, -6.7221) (13.0511, -6.7235) (13.0552, -6.7249) (13.0595, -6.7264) (13.0638, -6.7278) (13.0681, -6.7292) (13.0725, -6.7307) (13.0769, -6.7321) (13.0814, -6.7336) (13.0859, -6.7351) (13.0905, -6.7366) (13.0951, -6.738) (13.0998, -6.7395) (13.1046, -6.741) (13.1093, -6.7425) (13.1142, -6.744) (13.119, -6.7455) (13.124, -6.747) (13.1289, -6.7485) (13.1339, -6.75) (13.139, -6.7516) (13.1441, -6.7531) (13.1493, -6.7546) (13.1545, -6.7561) (13.1597, -6.7577) (13.165, -6.7592) (13.1704, -6.7607) (13.1758, -6.7623) (13.1812, -6.7638) (13.1867, -6.7653) (13.1922, -6.7669) (13.1978, -6.7684) (13.2034, -6.77) (13.209, -6.7715) (13.2147, -6.7731) (13.2205, -6.7746) (13.2263, -6.7761) (13.2321, -6.7777) (13.238, -6.7792) (13.2439, -6.7808) (13.2499, -6.7823) (13.2559, -6.7839) (13.2619, -6.7854) (13.268, -6.7869) (13.2742, -6.7885) (13.2804, -6.79) (13.2866, -6.7915) (13.2928, -6.7931) (13.2991, -6.7946) (13.3055, -6.7961) (13.3119, -6.7976) (13.3183, -6.7992) (13.3248, -6.8007) (13.3313, -6.8022) (13.3379, -6.8037) (13.3445, -6.8052) (13.3511, -6.8067) (13.3578, -6.8082) (13.3645, -6.8097) (13.3712, -6.8112) (13.378, -6.8127) (13.3849, -6.8142) (13.3918, -6.8157) (13.3987, -6.8171) (13.4056, -6.8186) (13.4126, -6.8201) (13.4197, -6.8215) (13.4267, -6.823) (13.4339, -6.8244) (13.441, -6.8259) (13.4482, -6.8273) (13.4554, -6.8288) (13.4627, -6.8302) (13.47, -6.8316) (13.4773, -6.833) (13.4847, -6.8344) (13.4922, -6.8358) (13.4996, -6.8372) (13.5071, -6.8386) (13.5146, -6.84) (13.5222, -6.8414) (13.5298, -6.8427) (13.5375, -6.8441) (13.5451, -6.8454) (13.5528, -6.8468) (13.5606, -6.8481) (13.5684, -6.8494) (13.5762, -6.8508) (13.5841, -6.8521) (13.592, -6.8534) (13.5999, -6.8547) (13.6079, -6.856) (13.6159, -6.8572) (13.6239, -6.8585) (13.632, -6.8598) (13.6401, -6.861) (13.6483, -6.8623) (13.6564, -6.8635) (13.6647, -6.8647) (13.6729, -6.8659) (13.6812, -6.8671) (13.6895, -6.8683) (13.6979, -6.8695) (13.7063, -6.8707) (13.7147, -6.8718) (13.7231, -6.873) (13.7316, -6.8741) (13.7401, -6.8753) (13.7487, -6.8764) (13.7573, -6.8775) (13.7659, -6.8786) (13.7746, -6.8797) (13.7833, -6.8808) (13.792, -6.8818) (13.8007, -6.8829) (13.8095, -6.884) (13.8184, -6.885) (13.8272, -6.886) (13.8361, -6.887) (13.845, -6.888) (13.854, -6.889) (13.8629, -6.89) (13.872, -6.891) (13.881, -6.8919) (13.8901, -6.8929) (13.8992, -6.8938) (13.9083, -6.8947) (13.9175, -6.8956) (13.9267, -6.8965) (13.936, -6.8974) (13.9452, -6.8982) (13.9545, -6.8991) (13.9639, -6.8999) (13.9732, -6.9008) (13.9826, -6.9016) (13.992, -6.9024) (14.0015, -6.9032) (14.011, -6.9039) (14.0205, -6.9047) (14.03, -6.9055) (14.0396, -6.9062) (14.0492, -6.9069) (14.0588, -6.9076) (14.0685, -6.9083) (14.0782, -6.909) (14.0879, -6.9097) (14.0976, -6.9103) (14.1074, -6.9109) (14.1172, -6.9116) (14.1271, -6.9122) (14.1369, -6.9128) (14.1468, -6.9134) (14.1568, -6.9139) (14.1667, -6.9145) (14.1767, -6.915) (14.1867, -6.9155) (14.1967, -6.916) (14.2068, -6.9165) (14.2169, -6.917) (14.227, -6.9175) (14.2372, -6.9179) (14.2474, -6.9183) (14.2576, -6.9188) (14.2678, -6.9192) (14.2781, -6.9195) (14.2883, -6.9199) (14.2987, -6.9203) (14.309, -6.9206) (14.3194, -6.9209) (14.3298, -6.9212) (14.3402, -6.9215) (14.3507, -6.9218) (14.3611, -6.9221) (14.3716, -6.9223) (14.3822, -6.9225) (14.3927, -6.9227) (14.4033, -6.9229) (14.4118, -6.9231) (14.4182, -6.9232) (14.4224, -6.9232) (14.4246, -6.9233) knots 0 0 0 0 0 0 0.00416667 0.00833333 0.0125 0.01666667 0.02083333 0.025 0.02916667 0.03333333 0.0375 0.04166667 0.04583333 0.05 0.05416667 0.05833333 0.0625 0.06666667 0.07083333 0.075 0.07916667 0.08333333 0.0875 0.09166667 0.09583333 0.1 0.10416667 0.10833333 0.1125 0.11666667 0.12083333 0.125 0.12916667 0.13333333 0.1375 0.14166667 0.14583333 0.15 0.15416667 0.15833333 0.1625 0.16666667 0.17083333 0.175 0.17916667 0.18333333 0.1875 0.19166667 0.19583333 0.2 0.20416667 0.20833333 0.2125 0.21666667 0.22083333 0.225 0.22916667 0.23333333 0.2375 0.24166667 0.24583333 0.25 0.25416667 0.25833333 0.2625 0.26666667 0.27083333 0.275 0.27916667 0.28333333 0.2875 0.29166667 0.29583333 0.3 0.30416667 0.30833333 0.3125 0.31666667 0.32083333 0.325 0.32916667 0.33333333 0.3375 0.34166667 0.34583333 0.35 0.35416667 0.35833333 0.3625 0.36666667 0.37083333 0.375 0.37916667 0.38333333 0.3875 0.39166667 0.39583333 0.4 0.40416667 0.40833333 0.4125 0.41666667 0.42083333 0.425 0.42916667 0.43333333 0.4375 0.44166667 0.44583333 0.45 0.45416667 0.45833333 0.4625 0.46666667 0.47083333 0.475 0.47916667 0.48333333 0.4875 0.49166667 0.49583333 0.5 0.50416667 0.50833333 0.5125 0.51666667 0.52083333 0.525 0.52916667 0.53333333 0.5375 0.54166667 0.54583333 0.55 0.55416667 0.55833333 0.5625 0.56666667 0.57083333 0.575 0.57916667 0.58333333 0.5875 0.59166667 0.59583333 0.6 0.60416667 0.60833333 0.6125 0.61666667 0.62083333 0.625 0.62916667 0.63333333 0.6375 0.64166667 0.64583333 0.65 0.65416667 0.65833333 0.6625 0.66666667 0.67083333 0.675 0.67916667 0.68333333 0.6875 0.69166667 0.69583333 0.7 0.70416667 0.70833333 0.7125 0.71666667 0.72083333 0.725 0.72916667 0.73333333 0.7375 0.74166667 0.74583333 0.75 0.75416667 0.75833333 0.7625 0.76666667 0.77083333 0.775 0.77916667 0.78333333 0.7875 0.79166667 0.79583333 0.8 0.80416667 0.80833333 0.8125 0.81666667 0.82083333 0.825 0.82916667 0.83333333 0.8375 0.84166667 0.84583333 0.85 0.85416667 0.85833333 0.8625 0.86666667 0.87083333 0.875 0.87916667 0.88333333 0.8875 0.89166667 0.89583333 0.9 0.90416667 0.90833333 0.9125 0.91666667 0.92083333 0.925 0.92916667 0.93333333 0.9375 0.94166667 0.94583333 0.95 0.95416667 0.95833333 0.9625 0.96666667 0.97083333 0.975 0.97916667 0.98333333 0.9875 0.99166667 0.99583333 1 1 1 1 1 1
  line L54 (12.9026, -6.6646) -> (12.9032, -6.6649)
  line L55 (-12.9026, -6.6646) -> (-12.2165, -6.3102)
  line L56 (12.223, -7.8417) -> (11.5731, -7.4247)
  line L57 (12.2236, -7.8421) -> (12.223, -7.8417)
  line L58 (10.326, -10.2121) -> (10.3255, -10.2117)
  line L59 (-3.681, -14.0486) -> (-3.6808, -14.048)
  line L60 (-5.2794, -13.5286) -> (-5.2796, -13.5292)
  line L61 (-6.5211, -12.9757) -> (-6.1743, -12.2858)
  line L62 (-6.5214, -12.9763) -> (-6.5211, -12.9757)
  line L63 (-3.6808, -14.048) -> (-3.4851, -13.301)
  line L64 (13.5863, 5.129) -> (13.5869, 5.1293)
  line L65 (-4.9987, -12.8092) -> (-5.2794, -13.5286)
  spline S30 degree 5 poles (15.9935, 0.4577) (15.9915, 0.4585) (15.9876, 0.4602) (15.9817, 0.4627) (15.9739, 0.466) (15.9641, 0.4702) (15.9544, 0.4743) (15.9447, 0.4784) (15.935, 0.4824) (15.9253, 0.4864) (15.9157, 0.4904) (15.906, 0.4944) (15.8964, 0.4984) (15.8868, 0.5023) (15.8772, 0.5062) (15.8676, 0.5101) (15.8581, 0.5139) (15.8486, 0.5177) (15.839, 0.5215) (15.8295, 0.5253) (15.8201, 0.529) (15.8106, 0.5328) (15.8012, 0.5365) (15.7918, 0.5401) (15.7824, 0.5438) (15.773, 0.5474) (15.7636, 0.551) (15.7543, 0.5546) (15.745, 0.5581) (15.7357, 0.5616) (15.7264, 0.5651) (15.7172, 0.5686) (15.7079, 0.572) (15.6987, 0.5755) (15.6895, 0.5789) (15.6803, 0.5822) (15.6712, 0.5856) (15.6621, 0.5889) (15.653, 0.5922) (15.6439, 0.5955) (15.6348, 0.5987) (15.6258, 0.6019) (15.6167, 0.6051) (15.6077, 0.6083) (15.5988, 0.6114) (15.5898, 0.6146) (15.5809, 0.6177) (15.572, 0.6207) (15.5631, 0.6238) (15.5542, 0.6268) (15.5454, 0.6298) (15.5365, 0.6328) (15.5278, 0.6358) (15.519, 0.6387) (15.5102, 0.6416) (15.5015, 0.6445) (15.4928, 0.6473) (15.4841, 0.6502) (15.4755, 0.653) (15.4668, 0.6558) (15.4582, 0.6585) (15.4497, 0.6613) (15.4411, 0.664) (15.4326, 0.6667) (15.4241, 0.6693) (15.4156, 0.672) (15.4071, 0.6746) (15.3987, 0.6772) (15.3903, 0.6797) (15.3819, 0.6823) (15.3736, 0.6848) (15.3652, 0.6873) (15.3569, 0.6898) (15.3487, 0.6923) (15.3404, 0.6947) (15.3322, 0.6971) (15.324, 0.6995) (15.3158, 0.7018) (15.3077, 0.7042) (15.2996, 0.7065) (15.2915, 0.7088) (15.2834, 0.7111) (15.2754, 0.7133) (15.2674, 0.7155) (15.2594, 0.7177) (15.2515, 0.7199) (15.2436, 0.7221) (15.2357, 0.7242) (15.2278, 0.7263) (15.22, 0.7284) (15.2122, 0.7305) (15.2044, 0.7325) (15.1967, 0.7345) (15.1889, 0.7365) (15.1813, 0.7385) (15.1736, 0.7405) (15.166, 0.7424) (15.1584, 0.7443) (15.1508, 0.7462) (15.1433, 0.7481) (15.1358, 0.7499) (15.1283, 0.7517) (15.1209, 0.7535) (15.1135, 0.7553) (15.1061, 0.7571) (15.0987, 0.7588) (15.0914, 0.7605) (15.0841, 0.7622) (15.0769, 0.7639) (15.0697, 0.7656) (15.0625, 0.7672) (15.0553, 0.7688) (15.0482, 0.7704) (15.0411, 0.772) (15.0341, 0.7735) (15.027, 0.775) (15.02, 0.7766) (15.0131, 0.778) (15.0062, 0.7795) (14.9993, 0.781) (14.9924, 0.7824) (14.9856, 0.7838) (14.9788, 0.7852) (14.9721, 0.7865) (14.9654, 0.7879) (14.9587, 0.7892) (14.9521, 0.7905) (14.9455, 0.7918) (14.9389, 0.7931) (14.9324, 0.7943) (14.9259, 0.7955) (14.9194, 0.7967) (14.913, 0.7979) (14.9066, 0.7991) (14.9003, 0.8002) (14.8939, 0.8014) (14.8877, 0.8025) (14.8814, 0.8036) (14.8753, 0.8047) (14.8691, 0.8057) (14.863, 0.8067) (14.8569, 0.8078) (14.8509, 0.8088) (14.8449, 0.8097) (14.8389, 0.8107) (14.833, 0.8117) (14.8271, 0.8126) (14.8213, 0.8135) (14.8155, 0.8144) (14.8097, 0.8153) (14.804, 0.8161) (14.7983, 0.817) (14.7927, 0.8178) (14.7871, 0.8186) (14.7816, 0.8194) (14.7761, 0.8201) (14.7706, 0.8209) (14.7652, 0.8216) (14.7598, 0.8224) (14.7545, 0.8231) (14.7492, 0.8237) (14.7439, 0.8244) (14.7387, 0.8251) (14.7336, 0.8257) (14.7285, 0.8263) (14.7234, 0.8269) (14.7184, 0.8275) (14.7134, 0.8281) (14.7085, 0.8287) (14.7036, 0.8292) (14.6988, 0.8298) (14.694, 0.8303) (14.6893, 0.8308) (14.6846, 0.8313) (14.6799, 0.8317) (14.6753, 0.8322) (14.6708, 0.8326) (14.6663, 0.8331) (14.6618, 0.8335) (14.6574, 0.8339) (14.6531, 0.8343) (14.6488, 0.8347) (14.6446, 0.835) (14.6404, 0.8354) (14.6362, 0.8357) (14.6321, 0.836) (14.6281, 0.8363) (14.6241, 0.8366) (14.6202, 0.8369) (14.6163, 0.8372) (14.6124, 0.8375) (14.6087, 0.8377) (14.605, 0.838) (14.6013, 0.8382) (14.5977, 0.8384) (14.5941, 0.8386) (14.5906, 0.8388) (14.5872, 0.839) (14.5838, 0.8392) (14.5805, 0.8393) (14.5772, 0.8395) (14.574, 0.8396) (14.5708, 0.8398) (14.5677, 0.8399) (14.5647, 0.84) (14.5617, 0.8401) (14.5588, 0.8402) (14.556, 0.8403) (14.5532, 0.8404) (14.5504, 0.8405) (14.5478, 0.8406) (14.5452, 0.8406) (14.5426, 0.8407) (14.5401, 0.8407) (14.5377, 0.8408) (14.5354, 0.8408) (14.5331, 0.8408) (14.5309, 0.8409) (14.5287, 0.8409) (14.5266, 0.8409) (14.5246, 0.8409) (14.5226, 0.8409) (14.5208, 0.8409) (14.519, 0.8409) (14.5172, 0.8409) (14.5155, 0.8409) (14.5139, 0.8409) (14.5124, 0.8408) (14.5109, 0.8408) (14.5096, 0.8408) (14.5082, 0.8408) (14.507, 0.8407) (14.5058, 0.8407) (14.5048, 0.8407) (14.5037, 0.8407) (14.5028, 0.8406) (14.502, 0.8406) (14.5012, 0.8406) (14.5005, 0.8406) (14.4999, 0.8405) (14.4993, 0.8405) (14.499, 0.8405) (14.4987, 0.8405) (14.4986, 0.8405) (14.4985, 0.8405) knots -1 -1 -1 -1 -1 -1 -0.99583333 -0.99166667 -0.9875 -0.98333333 -0.97916667 -0.975 -0.97083333 -0.96666667 -0.9625 -0.95833333 -0.95416667 -0.95 -0.94583333 -0.94166667 -0.9375 -0.93333333 -0.92916667 -0.925 -0.92083333 -0.91666667 -0.9125 -0.90833333 -0.90416667 -0.9 -0.89583333 -0.89166667 -0.8875 -0.88333333 -0.87916667 -0.875 -0.87083333 -0.86666667 -0.8625 -0.85833333 -0.85416667 -0.85 -0.84583333 -0.84166667 -0.8375 -0.83333333 -0.82916667 -0.825 -0.82083333 -0.81666667 -0.8125 -0.80833333 -0.80416667 -0.8 -0.79583333 -0.79166667 -0.7875 -0.78333333 -0.77916667 -0.775 -0.77083333 -0.76666667 -0.7625 -0.75833333 -0.75416667 -0.75 -0.74583333 -0.74166667 -0.7375 -0.73333333 -0.72916667 -0.725 -0.72083333 -0.71666667 -0.7125 -0.70833333 -0.70416667 -0.7 -0.69583333 -0.69166667 -0.6875 -0.68333333 -0.67916667 -0.675 -0.67083333 -0.66666667 -0.6625 -0.65833333 -0.65416667 -0.65 -0.64583333 -0.64166667 -0.6375 -0.63333333 -0.62916667 -0.625 -0.62083333 -0.61666667 -0.6125 -0.60833333 -0.60416667 -0.6 -0.59583333 -0.59166667 -0.5875 -0.58333333 -0.57916667 -0.575 -0.57083333 -0.56666667 -0.5625 -0.55833333 -0.55416667 -0.55 -0.54583333 -0.54166667 -0.5375 -0.53333333 -0.52916667 -0.525 -0.52083333 -0.51666667 -0.5125 -0.50833333 -0.50416667 -0.5 -0.49583333 -0.49166667 -0.4875 -0.48333333 -0.47916667 -0.475 -0.47083333 -0.46666667 -0.4625 -0.45833333 -0.45416667 -0.45 -0.44583333 -0.44166667 -0.4375 -0.43333333 -0.42916667 -0.425 -0.42083333 -0.41666667 -0.4125 -0.40833333 -0.40416667 -0.4 -0.39583333 -0.39166667 -0.3875 -0.38333333 -0.37916667 -0.375 -0.37083333 -0.36666667 -0.3625 -0.35833333 -0.35416667 -0.35 -0.34583333 -0.34166667 -0.3375 -0.33333333 -0.32916667 -0.325 -0.32083333 -0.31666667 -0.3125 -0.30833333 -0.30416667 -0.3 -0.29583333 -0.29166667 -0.2875 -0.28333333 -0.27916667 -0.275 -0.27083333 -0.26666667 -0.2625 -0.25833333 -0.25416667 -0.25 -0.24583333 -0.24166667 -0.2375 -0.23333333 -0.22916667 -0.225 -0.22083333 -0.21666667 -0.2125 -0.20833333 -0.20416667 -0.2 -0.19583333 -0.19166667 -0.1875 -0.18333333 -0.17916667 -0.175 -0.17083333 -0.16666667 -0.1625 -0.15833333 -0.15416667 -0.15 -0.14583333 -0.14166667 -0.1375 -0.13333333 -0.12916667 -0.125 -0.12083333 -0.11666667 -0.1125 -0.10833333 -0.10416667 -0.1 -0.09583333 -0.09166667 -0.0875 -0.08333333 -0.07916667 -0.075 -0.07083333 -0.06666667 -0.0625 -0.05833333 -0.05416667 -0.05 -0.04583333 -0.04166667 -0.0375 -0.03333333 -0.02916667 -0.025 -0.02083333 -0.01666667 -0.0125 -0.00833333 -0.00416667 0 0 0 0 0 0
  arc A43 (15.9935, -0.4577) -> (15.9935, 0.4577) centre (0, 0) ccw
  line L66 (14.4979, 0.8404) -> (13.727, 0.7957)
  line L67 (-0.6796, -14.5069) -> (-0.6796, -14.5063)